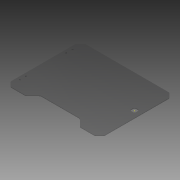
# Autodesk Inventor part: D-049
Saved by Autodesk Inventor 2015 (Build 190159000, 159)
## iProperties
Company: MARCHA TECHNOLOGY
Created: 2013-10-01
Part Number: D-049
Document SubType Name: Modeling
Designer: O.Martin
Density: 1 g/cm^3
Project: WITBOXprinter_K01
Description: PUERTA FRONTAL
Stock Number: 28655
Mass: 326.697 g
Surface Area: 2216.72 cm^2
Volume: 326.697 cm^3
Material: Generic
Appearance: Light Gray Reflective
Author: O.Martin
Autodesk Inventor part; units mm, degrees
ref_plane "YZ Plane" through (0, 0, 0) normal (1, 0, 0) x (0, 1, 0)
ref_plane "XZ Plane" through (0, 0, 0) normal (0, 1, 0) x (-1, 0, 0)
ref_plane "XY Plane" through (0, 0, 0) normal (0, 0, 1) x (1, 0, 0)
sketch "Boceto1" plane through (0, 0, 0) normal (0, 0, 1) x (1, 0, 0)
  circle A0 centre (-214, -182.25) radius 3.25 construction
  circle A1 centre (214, -182.25) radius 3.25 construction
  circle A2 centre (214, 182.25) radius 3.25 construction
  circle A3 centre (-214, 182.25) radius 3.25 construction
  line L0 (-240, 193.25) -> (-240, -193.25) construction
  line L1 (-223, 210.25) -> (-240, 193.25) construction
  line L2 (240, 193.25) -> (223, 210.25) construction
  line L3 (240, -193.25) -> (240, 193.25) construction
  line L4 (215, -218.25) -> (240, -193.25) construction
  line L5 (-215, -218.25) -> (215, -218.25) construction
  line L6 (-240, -193.25) -> (-215, -218.25) construction
  line L7 (-192.5, 116.75) -> (-209.5, 116.75) construction
  line L8 (-211.5, 114.75) -> (-211.5, 76.75) construction
  line L9 (-209.5, 74.75) -> (-192.5, 74.75) construction
  line L10 (-192.5, 74.75) -> (-192.5, -74.75) construction
  line L11 (-192.5, -74.75) -> (-209.5, -74.75) construction
  line L12 (-211.5, -76.75) -> (-211.5, -114.75) construction
  line L13 (-209.5, -116.75) -> (-192.5, -116.75) construction
  line L14 (-192.5, -116.75) -> (-192.5, -129.1079) construction
  arc A4 (-192.5, -129.1079) -> (-189.5711, -136.1789) centre (-182.5, -129.1079) ccw construction
  line L15 (-189.5711, -136.1789) -> (-175.4289, -150.3211) construction
  arc A5 (-175.4289, -150.3211) -> (-168.3579, -153.25) centre (-168.3579, -143.25) ccw construction
  line L16 (-168.3579, -153.25) -> (-114.1421, -153.25) construction
  arc A6 (192.5, 129.1079) -> (189.5711, 136.1789) centre (182.5, 129.1079) ccw construction
  line L17 (189.5711, 136.1789) -> (175.4289, 150.3211) construction
  arc A7 (175.4289, 150.3211) -> (168.3579, 153.25) centre (168.3579, 143.25) ccw construction
  line L18 (168.3579, 153.25) -> (-168.3579, 153.25) construction
  arc A8 (-168.3579, 153.25) -> (-175.4289, 150.3211) centre (-168.3579, 143.25) ccw construction
  line L19 (-175.4289, 150.3211) -> (-189.5711, 136.1789) construction
  arc A9 (-189.5711, 136.1789) -> (-192.5, 129.1079) centre (-182.5, 129.1079) ccw construction
  line L20 (-192.5, 129.1079) -> (-192.5, 116.75) construction
  line L21 (-49.5, -150.75) -> (-49.5, -188.75) construction
  arc A10 (-49.5, -188.75) -> (-47.5, -190.75) centre (-47.5, -188.75) ccw construction
  line L22 (-47.5, -190.75) -> (47.5, -190.75) construction
  arc A11 (47.5, -190.75) -> (49.5, -188.75) centre (47.5, -188.75) ccw construction
  line L23 (49.5, -188.75) -> (49.5, -150.75) construction
  arc A12 (49.5, -150.75) -> (47.5, -148.75) centre (47.5, -150.75) ccw construction
  line L24 (47.5, -148.75) -> (-47.5, -148.75) construction
  arc A13 (-47.5, -148.75) -> (-49.5, -150.75) centre (-47.5, -150.75) ccw construction
  circle A14 centre (73.4, -166.85) radius 6 construction
  arc A15 (-114.1421, -153.25) -> (-107.0711, -150.3211) centre (-114.1421, -143.25) ccw projected
  line L25 (-107.0711, -150.3211) -> (-82.9289, -126.1789) projected
  line L26 (-75.8579, -123.25) -> (75.8579, -123.25) projected
  line L27 (192.5, -129.1079) -> (192.5, 129.1079) projected
  arc A16 (-75.8579, -123.25) -> (-82.9289, -126.1789) centre (-75.8579, -133.25) ccw projected
  arc A17 (82.9289, -126.1789) -> (75.8579, -123.25) centre (75.8579, -133.25) ccw projected
  line L28 (82.9289, -126.1789) -> (107.0711, -150.3211) projected
  arc A18 (107.0711, -150.3211) -> (114.1421, -153.25) centre (114.1421, -143.25) ccw projected
  line L29 (114.1421, -153.25) -> (168.3579, -153.25) projected
  arc A19 (168.3579, -153.25) -> (175.4289, -150.3211) centre (168.3579, -143.25) ccw projected
  line L30 (175.4289, -150.3211) -> (189.5711, -136.1789) projected
  arc A20 (189.5711, -136.1789) -> (192.5, -129.1079) centre (182.5, -129.1079) ccw projected
  line L31 (-168.3579, 151.75) -> (168.3579, 151.75)
  arc A21 (174.3683, 149.2604) -> (168.3579, 151.75) centre (168.3579, 143.25) ccw
  line L32 (174.3683, 149.2604) -> (188.5104, 135.1183)
  arc A22 (191, 129.1079) -> (188.5104, 135.1183) centre (182.5, 129.1079) ccw
  line L33 (191, 129.1079) -> (191, -129.1079)
  arc A23 (188.5104, -135.1183) -> (191, -129.1079) centre (182.5, -129.1079) ccw
  line L34 (188.5104, -135.1183) -> (174.3683, -149.2604)
  arc A24 (168.3579, -151.75) -> (174.3683, -149.2604) centre (168.3579, -143.25) ccw
  line L35 (168.3579, -151.75) -> (114.1421, -151.75)
  arc A25 (108.1317, -149.2604) -> (114.1421, -151.75) centre (114.1421, -143.25) ccw
  line L36 (108.1317, -149.2604) -> (83.9896, -125.1183)
  arc A26 (83.9896, -125.1183) -> (75.8579, -121.75) centre (75.8579, -133.25) ccw
  line L37 (75.8579, -121.75) -> (-75.8579, -121.75)
  arc A27 (-75.8579, -121.75) -> (-83.9896, -125.1183) centre (-75.8579, -133.25) ccw
  line L38 (-83.9896, -125.1183) -> (-108.1317, -149.2604)
  arc A28 (-114.1421, -151.75) -> (-108.1317, -149.2604) centre (-114.1421, -143.25) ccw
  line L39 (-114.1421, -151.75) -> (-168.3579, -151.75)
  arc A29 (-174.3683, -149.2604) -> (-168.3579, -151.75) centre (-168.3579, -143.25) ccw
  line L40 (-174.3683, -149.2604) -> (-188.5104, -135.1183)
  arc A30 (-191, -129.1079) -> (-188.5104, -135.1183) centre (-182.5, -129.1079) ccw
  line L41 (-191, -129.1079) -> (-191, -115.25)
  line L42 (-191, -115.25) -> (-210, -115.25)
  line L43 (-210, -115.25) -> (-210, -76.25)
  line L44 (-210, -76.25) -> (-191, -76.25)
  line L45 (-191, -76.25) -> (-191, 76.25)
  line L46 (-191, 76.25) -> (-210, 76.25)
  line L47 (-210, 76.25) -> (-210, 115.25)
  line L48 (-210, 115.25) -> (-191, 115.25)
  line L49 (-191, 115.25) -> (-191, 129.1079)
  arc A31 (-188.5104, 135.1183) -> (-191, 129.1079) centre (-182.5, 129.1079) ccw
  line L50 (-188.5104, 135.1183) -> (-174.3683, 149.2604)
  arc A32 (-168.3579, 151.75) -> (-174.3683, 149.2604) centre (-168.3579, 143.25) ccw
  line L51 (-191, 115.25) -> (-191, 76.25)
  line L52 (-191, -76.25) -> (-191, -115.25)
  circle A33 centre (73.4, -148.15) radius 7.5 projected
  line L53 (-223, 210.25) -> (223, 210.25) projected
  arc A34 (-209.5, 116.75) -> (-211.5, 114.75) centre (-209.5, 114.75) ccw projected
  arc A35 (-211.5, 76.75) -> (-209.5, 74.75) centre (-209.5, 76.75) ccw projected
  arc A36 (-209.5, -74.75) -> (-211.5, -76.75) centre (-209.5, -76.75) ccw projected
  arc A37 (-211.5, -114.75) -> (-209.5, -116.75) centre (-209.5, -114.75) ccw projected
  dimension "d23" = 1.5
  constraints: 44 end point, 24 point on circle, 12 centre point, 2 collinear, 31 other
  measures "d23" distance between parallel lines of L18 L31
extrude "Extrusión1" add sketch "Boceto1" along normal blind 3 contours L31 A21 L32 A22 L33 A23 L34 A24 L35 A25 L36 A26 L37 A27 L38 A28 L39 A29 L40 A30 L41 L52 L45 L51 L49 A31 L50 A32
sketch "Boceto2" plane through (0, 0, 3) normal (0, 0, 1) x (1, 0, 0)
  line L0 (-178, 106.25) -> (-178, 81.25) construction
  line L1 (-178, -83.25) -> (-178, -108.25) construction
  line L2 (-191, -129.1079) -> (-191, 129.1079) projected
  line L3 (-114.1421, -151.75) -> (-168.3579, -151.75) projected
  dimension "d3" = 25
  dimension "d25" = 13
  dimension "d28" = 43.5
  dimension "d29" = 189.5
  constraints: 4 coincident, 4 end point, 2 collinear, 1 vertical alignment
  measures "d3" distance of L0.start L0.end
  measures "d25" distance between parallel lines of L0 L2
  measures "d28" distance from line of L3 point (-178, -108.25)
  measures "d29" distance of point (-178, -108.25) point (-178, 81.25)
hole "Agujero1" at (-178, 106.25, 3) at (-178, 81.25, 3) at (-178, -83.25, 3) at (-178, -108.25, 3) direction (0, 0, -1) diameter 5 end through all
chamfer "Chaflán1" distance 0.5 angle 45 48 edges at (-191, 0, 3) (-190.353, 132.3607, 3) (-181.4393, 142.1893, 3) (-171.6107, 151.103, 3) (0, 151.75, 3) (171.6107, 151.103, 3) (181.4393, 142.1893, 3) (190.353, 132.3607, 3) (191, 0, 3) (190.353, -132.3607, 3) (181.4393, -142.1893, 3) (171.6107, -151.103, 3) (141.25, -151.75, 3) (110.8893, -151.103, 3) (96.0607, -137.1893, 3) (80.2587, -122.6254, 3) (0, -121.75, 3) (-80.2587, -122.6254, 3) (-96.0607, -137.1893, 3) (-110.8893, -151.103, 3) (-141.25, -151.75, 3) (-171.6107, -151.103, 3) (-181.4393, -142.1893, 3) (-190.353, -132.3607, 3) (-181.4393, 142.1893, 0) (-190.353, 132.3607, 0) (-191, 0, 0) (-190.353, -132.3607, 0) (-181.4393, -142.1893, 0) (-171.6107, -151.103, 0) (-141.25, -151.75, 0) (-110.8893, -151.103, 0) (-96.0607, -137.1893, 0) (-80.2587, -122.6254, 0) (0, -121.75, 0) (80.2587, -122.6254, 0) (96.0607, -137.1893, 0) (110.8893, -151.103, 0) (141.25, -151.75, 0) (171.6107, -151.103, 0) (181.4393, -142.1893, 0) (190.353, -132.3607, 0) (191, 0, 0) (190.353, 132.3607, 0) (181.4393, 142.1893, 0) (171.6107, 151.103, 0) (0, 151.75, 0) (-171.6107, 151.103, 0)
sketch "Boceto3" plane through (0, 0, 3) normal (0, 0, 1) x (1, 0, 0)
  line L0 (153.45, 28.3) -> (173.55, 28.3)
  line L1 (173.55, 28.3) -> (173.55, 8.2)
  line L2 (173.55, 8.2) -> (153.45, 8.2)
  line L3 (153.45, 8.2) -> (153.45, 28.3)
  line L4 (153.45, 24.1099) -> (157.6401, 28.3)
  line L5 (169.3599, 28.3) -> (173.55, 24.1099)
  line L6 (173.55, 12.3901) -> (169.3599, 8.2)
  line L7 (157.6401, 8.2) -> (153.45, 12.3901)
  line L8 (153.45, 18.25) -> (173.55, 18.25) construction
  line L9 (163.5, 28.3) -> (163.5, 8.2) construction
  line L10 (168.3579, -151.25) -> (114.1421, -151.25) projected
  line L11 (190.5, 129.1079) -> (190.5, -129.1079) projected
  point P0 (163.5, 18.25)
  dimension "d17" = 20.1
  dimension "d18" = 22.5
  dimension "d26" = 169.5
  dimension "d27" = 27
  constraints: 20 end point, 8 perpendicular, 8 point on line, 5 midpoint, 2 parallel, 1 horizontal
  measures "d17" distance of L0.start L0.end
  measures "d18" distance between parallel lines of L7 L5
  measures "d26" distance between parallel lines of L10 L8
  measures "d27" distance between parallel lines of L11 L9
extrude "Extrusión2" cut sketch "Boceto3" against normal through all contours L0 L5 L1 L6 L2 L7 L3 L4
body "Solid1"
